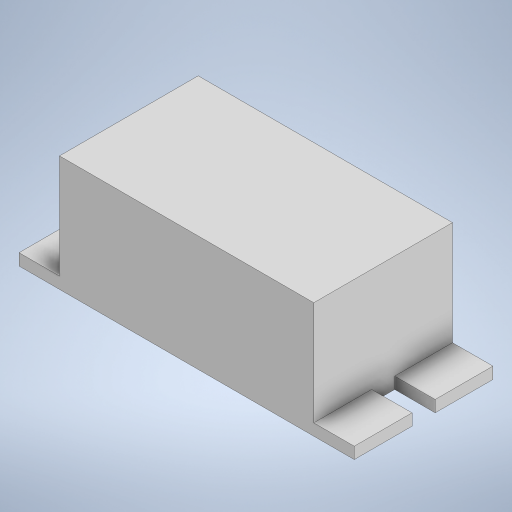
# Autodesk Inventor part: DCDC24Vto15V
Saved by Autodesk Inventor 2023 (Build 270158000, 158)
## iProperties
Created: 2023-10-03
Part Number: DCDC24Vto15V
Material: 一般
Document SubType Name: Modeling
Designer: 310611102
Density: 1 g/cm^3
Appearance: 預設
Author: 310611102
Autodesk Inventor part; units mm, degrees
ref_plane "YZ Plane" through (0, 0, 0) normal (1, 0, 0) x (0, 1, 0)
ref_plane "XZ Plane" through (0, 0, 0) normal (0, 1, 0) x (-1, 0, 0)
ref_plane "XY Plane" through (0, 0, 0) normal (0, 0, 1) x (1, 0, 0)
sketch "Sketch1" plane through (0, 0, 0) normal (0, 0, 1) x (1, 0, 0)
  line L0 (-22, 20) -> (22, 20)
  line L1 (22, 20) -> (22, 0)
  line L2 (22, 0) -> (-22, 0)
  line L3 (-22, 0) -> (-22, 20)
  line L4 (-22, 20) -> (22, 0) construction
  line L5 (22, 20) -> (-22, 0) construction
  line L6 (-29, 2) -> (-22, 2)
  line L7 (-22, 2) -> (-22, 0)
  line L8 (-22, 0) -> (-29, 0)
  line L9 (-29, 0) -> (-29, 2)
  line L10 (-29, 2) -> (-22, 0) construction
  line L11 (-22, 2) -> (-29, 0) construction
  line L12 (29, 2) -> (22, 2)
  line L13 (22, 2) -> (22, 0)
  line L14 (22, 0) -> (29, 0)
  line L15 (29, 0) -> (29, 2)
  line L16 (29, 2) -> (22, 0) construction
  line L17 (22, 2) -> (29, 0) construction
  point P0 (0, 0)
  point P1 (0, 10)
  point P2 (-25.5, 1)
  point P3 (25.5, 1)
  dimension "d0" = 58
  dimension "d1" = 20
  dimension "d2" = 2
  dimension "d3" = 44
  constraints: 36 end point, 7 midpoint, 6 parallel, 3 collinear, 3 horizontal, 3 perpendicular, 1 point on line, 1 vertical alignment
  measures "d0" distance between parallel lines of L15 L9
  measures "d1" distance between parallel lines of L2 L0
  measures "d2" distance between parallel lines of L14 L12
  measures "d3" distance of L0.start L0.end
extrude "Extrusion1" add sketch "Sketch1" along normal mid plane 24
sketch "Sketch2" plane through (-29, 0, 12) normal (0, -1, 0) x (1, 0, 0)
  line L0 (58, -24) -> (58, 0) projected
  line L1 (51, -10) -> (58, -10)
  line L2 (58, -10) -> (58, -14)
  line L3 (58, -14) -> (51, -14)
  line L4 (51, -14) -> (51, -10)
  line L5 (51, -10) -> (58, -14) construction
  line L6 (58, -10) -> (51, -14) construction
  line L7 (0, -24) -> (0, 0) projected
  line L8 (7, -10) -> (0, -10)
  line L9 (0, -10) -> (0, -14)
  line L10 (0, -14) -> (7, -14)
  line L11 (7, -14) -> (7, -10)
  line L12 (7, -10) -> (0, -14) construction
  line L13 (0, -10) -> (7, -14) construction
  point P0 (29, -12)
  point P1 (54.5, -12)
  point P2 (3.5, -12)
  point P3 (0, -10)
  dimension "d6" = 4
  dimension "d7" = 44
  constraints: 24 end point, 4 midpoint, 4 parallel, 3 point on line, 2 collinear, 2 horizontal, 2 perpendicular, 1 horizontal alignment
  measures "d6" distance of L3.end L1.start
  measures "d7" distance between parallel lines of L11 L4
extrude "Extrusion2" cut sketch "Sketch2" against normal blind 24
body "Solid1"
